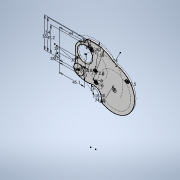
# Autodesk Inventor part: 足内フレーム
Saved by Autodesk Inventor 2022.2 (Build 262287010, 287A)
## iProperties
Created: 2022-01-10
Part Number: 足内フレーム
Material: Aluminum 2014-T4
Document SubType Name: Modeling
Designer: acps
Density: 2.8 g/cm^3
Appearance: Satin
Author: acps
Autodesk Inventor part; units mm, degrees
ref_plane "YZ Plane" through (0, 0, 0) normal (1, 0, 0) x (0, 1, 0)
ref_plane "XZ Plane" through (0, 0, 0) normal (0, 1, 0) x (-1, 0, 0)
ref_plane "XY Plane" through (0, 0, 0) normal (0, 0, 1) x (1, 0, 0)
sketch "Sketch2" plane through (0, 0, 0) normal (0, 0, 1) x (1, 0, 0)
  circle A0 centre (46.4683, 30) radius 14
  circle A1 centre (66.4734, 20) radius 20.5 construction
  circle A2 centre (100, 0) radius 30 construction
  circle A3 centre (123.045, 25) radius 3
  circle A4 centre (100, 0) radius 3
  circle A5 centre (35, 0) radius 1.5
  circle A6 centre (35, 0) radius 9
  arc A7 (26.7096, 3.5028) -> (28.8661, 26.2368) centre (-8.2942, 18.2924) ccw
  arc A8 (44, 47.83) -> (28.8661, 26.2368) centre (46.4683, 30) ccw
  arc A9 (110.626, 39.2116) -> (45.1112, 47.9488) centre (57.174, -111.5959) ccw construction
  arc A10 (91.0834, -36) -> (110.626, 39.2116) centre (97.597, 2.4523) ccw
  arc A11 (28.6833, 27.2278) -> (91.0834, -36) centre (103.7766, 38.9326) ccw construction
  circle A12 centre (58.3063, 43.4) radius 3
  arc A13 (44.5539, 47.9057) -> (44, 47.83) centre (65.9403, -110.6586) ccw
  arc A14 (58.162, 47.5669) -> (44.5539, 47.9057) centre (50.3015, 5.2915) ccw construction
  arc A15 (91.0834, -36) -> (110.626, 39.2116) centre (97.597, 2.4523) ccw
  arc A16 (75.5201, -28.3291) -> (58.8706, -11.0424) centre (62.0019, -24.6878) ccw
  arc A17 (31.2271, -8.171) -> (58.8706, -11.0424) centre (49.2531, 30.8682) ccw
  arc A18 (75.5201, -28.3291) -> (76.4189, -30.5623) centre (77.4512, -28.8493) ccw
  arc A19 (76.4189, -30.5623) -> (91.0834, -36) centre (98.0981, 5.4101) ccw
  circle A20 centre (58.3063, 43.4) radius 3 construction
  circle A21 centre (123.045, 25) radius 3
  circle A22 centre (100, 0) radius 3
  circle A23 centre (65.359, 13) radius 3
  circle A24 centre (66.299, -4.4994) radius 4 construction
  circle A25 centre (66.299, -4.4994) radius 3
  circle A26 centre (66.299, -4.4994) radius 1.5
  circle A27 centre (58.3063, 43.4) radius 1.5
  circle A28 centre (53.0056, 45.2) radius 1.25
  arc A29 (68.5309, 40.8961) -> (47.0781, 45.1614) centre (50.3015, 5.2915) ccw construction
  circle A30 centre (45.1, 8.5) radius 1.25
  circle A31 centre (33, 18) radius 1.25
  line L0 (35, 0) -> (22.7472, 0) construction
  arc A32 (110.5809, -8.3302) -> (32.9301, 51.0574) centre (65.359, 13) ccw construction
  arc A33 (96.7545, 45.0877) -> (104.0739, 41.376) centre (111.1088, 64.3218) ccw
  arc A34 (110.626, 39.2116) -> (104.0739, 41.376) centre (57.174, -111.5959) ccw
  arc A35 (44.5539, 47.9057) -> (47.2438, 50.582) centre (44.1342, 51.0175) ccw
  arc A36 (52.2805, 55.7739) -> (47.2438, 50.582) centre (53.3146, 49.7317) ccw
  arc A37 (96.7545, 45.0877) -> (52.2805, 55.7739) centre (62.0648, -1.3949) ccw
  circle A38 centre (65.359, 13) radius 1.25
  circle A39 centre (123.045, 25) radius 1.25
  point P0 (0, 0)
  point P1 (48.9147, 54)
  point P2 (75.6154, 55)
  dimension "d120" = 3
  dimension "d121" = 18
  dimension "d122" = 4
  dimension "d123" = 38
  dimension "d124" = 14
  dimension "d125" = 2
  dimension "d126" = 43
  dimension "d127" = 43
  dimension "d129" = 44
  dimension "d130" = 42
  dimension "d131" = 74
  dimension "d132" = 118
  dimension "d133" = 6
  dimension "d134" = 8
  dimension "d135" = 6
  dimension "d136" = 3
  dimension "d137" = 3
  dimension "d138" = 2.5
  dimension "d139" = 3
  dimension "d140" = 2.5
  dimension "d141" = 45.2
  dimension "d142" = 8.5
  dimension "d143" = 45.1
  dimension "d144" = 2.5
  dimension "d145" = 35
  dimension "d146" = 18
  dimension "d147" = 33
  dimension "d148" = 50
  dimension "d149" = 3.14
  dimension "d150" = 6.13
  dimension "d151" = 58
  dimension "d152" = 24
  dimension "d153" = 54
  dimension "d154" = 55
  dimension "d160" = 2.5
  dimension "d161" = 2.5
  constraints: 41 point on circle, 39 centre point, 17 tangent, 10 coincident, 6 concentric, 2 end point, 2 horizontal, 19 other
  measures "d120" diameter of A5
  measures "d121" diameter of A6
  measures "d122" radial gap between concentric circles of A8 A0
  measures "d123" radius of A7
  measures "d124" radius of A16
  measures "d125" radius of A18
  measures "d126" radius of A17
  measures "d127" radius of A14
  measures "d129" horizontal distance of point (0, 0) A8.start
  measures "d130" radius of A19
  measures "d133" diameter of A23
  measures "d134" diameter of A24
  measures "d135" diameter of A25
  measures "d136" diameter of A26
  measures "d137" diameter of A27
  measures "d138" diameter of A28
  measures "d139" radial gap between concentric circles of A14 A29
  measures "d140" diameter of A30
  measures "d141" vertical distance of point (0, 0) A28.centre
  measures "d142" vertical distance of point (0, 0) A30.centre
  measures "d143" horizontal distance of point (0, 0) A30.centre
  measures "d144" diameter of A31
  measures "d145" distance of point (0, 0) A5.centre
  measures "d146" vertical distance of point (0, 0) A31.centre
  measures "d147" horizontal distance of point (0, 0) A31.centre
  measures "d148" radius of A32
  measures "d149" radius of A35
  measures "d150" radius of A36
  measures "d151" radius of A37
  measures "d152" radius of A33
  measures "d153" vertical distance of point (0, 0) point (48.915, 54)
  measures "d154" vertical distance of point (0, 0) point (75.615, 55)
  measures "d160" diameter of A38
  measures "d161" diameter of A39
extrude "Extrusion1" add sketch "Sketch2" against normal blind 3 contours A3 | A6 | A6 A7 A8 A13 A35 A36 A37 A33 A34 A10 A19 A18 A16 A17 | A12 | A23 | A25
sketch "export" plane through (0, 0, 0) normal (0, 0, 1) x (1, 0, 0)
  circle A0 centre (123.045, 25) radius 3 projected
  circle A1 centre (65.359, 13) radius 3 projected
  circle A2 centre (65.359, 13) radius 1.25 projected
  circle A3 centre (58.3063, 43.4) radius 1.5 projected
  circle A4 centre (123.045, 25) radius 1.25 projected
  point P0 (0, 0)
extrude "Extrusion2" cut sketch "Sketch2" against normal blind 1 contours A3 | A12 | A23 | A25
body "Solid1"
